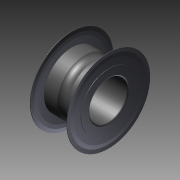
# Autodesk Inventor part: W 638/4 XR-2Z_PART1
Saved by Autodesk Inventor 2011 SP1 (Build 150282100, 282)
## iProperties
Created: 2017-05-31
Part Number: W 638/4 XR-2Z_PART1
Catalog Web Link: www.cadenas.de
Description: -Deep groove ball bearings, stainless steel, single row, with flanged outer ring
Vendor: SKF
Document SubType Name: Modeling
Designer: psAdmin
Manufacturer: SKF
Mass: 0.0609967 g
Surface Area: 2.88206 cm^2
Volume: 0.0609967 cm^3
Density: 1 g/cm^3
Category: PARTsolutions
Company: SKF
Title: W 638/4 XR-2Z_PART1
Author: Cadenas PARTsolutions
Comments: Deep groove ball bearings, stainless steel, single row, with flanged outer ring
PSOL_IDENT_0: {$CADENAS_DATA\23d-libs\skf\bearings_units_and_housings\ball_bearings\deep_groove_ball_bearings\deep
PSOL_IDENT_1: _groove_ball_bearings_stainless_steel\bb1_005_105.prj},207 {VTYP=3D},{NB=W 638/4 XR-2Z_PART1},{LINA=
PSOL_IDENT_2: W 638/4 XR-2Z_PART1},{NN=BB1_005_105_PART1},{NOPRJ=TRUE},{DATE=12.09.2016 08:57:11},{GEOMDATE=26.04.
PSOL_IDENT_3: 2016 08:41:00},{VERSION=},{LINEID=51210},{LINESUBID=-1},{WBVAR=}  {NB=W 638/4 XR-2Z_PART1},{LINA=W 6
PSOL_IDENT_4: 38/4 XR-2Z_PART1},{KT=DUMMY},{PRODUCTID=},{DESIGNATION=W 638/4 XR-2Z},{DD=4.000},{D=10.000},{B=4.000
PSOL_IDENT_5: },{C=0.800},{DD1=5.900},{DD2=-1000000015047466219876688855040.000},{D1=8.200},{D2=8.800},{D3=11.600}
PSOL_IDENT_6: ,{R12=0.150},{LOAD1=0.553},{LOAD2=0.245},{LOAD3=0.011},{SPEED1=130000},{SPEED2=63000},{MASS=0.0015},
PSOL_IDENT_7: {PITCH=7.100},{DW=1.588},{Z=8.000},{II=1.000},{TYPEID=-1000000015047466219876688855040},{DESIGN=dgbb
PSOL_IDENT_8: wr2z},{MAPPING=BCZ50,DESIGNATION|IRD01,DD|ORD10,D|BCW30,B|ORL02,C|IRD30,DD1|ORD30,D1|IRD43,DD2|ORD43
PSOL_IDENT_9: ,D2|ORD15,D3|ORR20,R12|BCC02,LOAD1|BCC16,LOAD2|BCC12,LOAD3|BCC43,SPEED1|BCC45,SPEED2|BCM01,MASS|BCD5
PSOL_IDENT_10: 0,PITCH|RBD10,DW|BCN81,Z|BCN80,II},{DESIGNLIST=dgbbwr2rs,dgbbwr,dgbbwr2z,dgbbwr2rz,dgbbwr2zs},{SORT=
PSOL_IDENT_11: DD},{SH=5.9},{PIM=W 638/4 XR-2Z}
NT: Deep groove ball bearings, stainless steel, single row, with flanged outer ring
NB: W 638/4 XR-2Z_PART1
NBSYN: $DESIGNATION._PART1
LINA: W 638/4 XR-2Z_PART1
DESIGNATION: W 638/4 XR-2Z
DD: 4.000
D: 10.000
B: 4.000
LOAD1: 0.553
LOAD2: 0.245
LOAD3: 0.011
SPEED1: 130000
SPEED2: 63000
SUPPLIER: SKF
ARTICLENO: W 638/4 XR-2Z_PART1
BOMINFO: W 638/4 XR-2Z_PART1
CREATOR: CADENAS GmbH
Autodesk Inventor part; units mm, degrees
ref_plane "YZ Plane" through (0, 0, 0) normal (1, 0, 0) x (0, 1, 0)
ref_plane "XZ Plane" through (0, 0, 0) normal (0, 1, 0) x (-1, 0, 0)
ref_plane "XY Plane" through (0, 0, 0) normal (0, 0, 1) x (1, 0, 0)
sketch "Sketch_13" plane through (0, 0, 0) normal (0, 0, 1) x (1, 0, 0)
  line L0 (2, 0) -> (-2, 0)
  arc A0 (0, 2.15) -> (0.15, 2) centre (0.15, 2.15) ccw
  line L1 (0.15, 2) -> (3.85, 2)
  arc A1 (3.85, 2) -> (4, 2.15) centre (3.85, 2.15) ccw
  line L2 (4, 2.15) -> (4, 2.95)
  line L3 (4, 2.95) -> (2.52, 2.95)
  arc A2 (1.48, 2.95) -> (2.52, 2.95) centre (2, 3.55) ccw
  line L4 (1.48, 2.95) -> (0, 2.95)
  line L5 (0, 2.95) -> (0, 2.15)
  constraints: 12 end point, 6 point on circle, 3 centre point
revolve "Revolution1" add sketch "Sketch_13" angle 360 about axis through (2, 0, 0) along (1, 0, 0)
sketch "Sketch_25" plane through (0, 0, 0) normal (0, 0, 1) x (1, 0, 0)
  line L0 (50, 0) -> (-50, 0)
  line L1 (0.0375, 4.4) -> (0.06, 4.0375)
  line L2 (0.06, 4.0375) -> (0.0375, 3.675)
  line L3 (0.0375, 3.675) -> (0.0375, 2.95)
  line L4 (0.0375, 2.95) -> (0.0825, 2.95)
  line L5 (0.0825, 2.95) -> (0.1275, 3.675)
  line L6 (0.1275, 3.675) -> (0.1275, 4.0375)
  line L7 (0.1275, 4.0375) -> (0.0825, 4.4)
  line L8 (0.0825, 4.4) -> (0.0375, 4.4)
  constraints: 18 end point
revolve "Revolution2" add sketch "Sketch_25" angle 360 about axis through (50, 0, 0) along (1, 0, 0)
sketch "Sketch_26" plane through (0, 0, 0) normal (0, 0, 1) x (1, 0, 0)
  line L0 (50, 0) -> (-50, 0)
  line L1 (3.8725, 4.0375) -> (3.8725, 3.675)
  line L2 (3.8725, 3.675) -> (3.9175, 2.95)
  line L3 (3.9175, 2.95) -> (3.9625, 2.95)
  line L4 (3.9625, 2.95) -> (3.9625, 3.675)
  line L5 (3.9625, 3.675) -> (3.94, 4.0375)
  line L6 (3.94, 4.0375) -> (3.9625, 4.4)
  line L7 (3.9625, 4.4) -> (3.9175, 4.4)
  line L8 (3.9175, 4.4) -> (3.8725, 4.0375)
  constraints: 18 end point
revolve "Revolution3" add sketch "Sketch_26" angle 360 about axis through (50, 0, 0) along (1, 0, 0)
body "Solid1"
